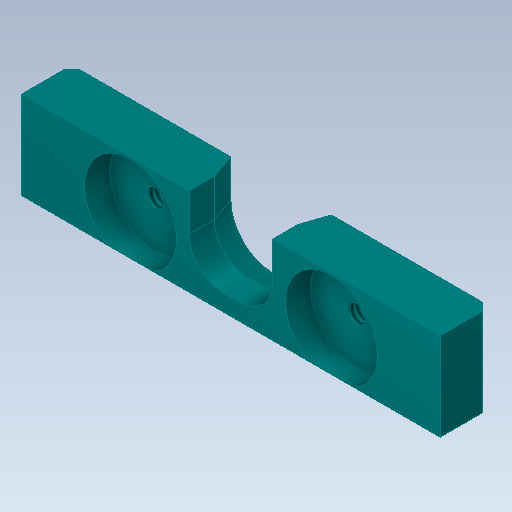
# Autodesk Inventor part: FAB-OX0021
Saved by Autodesk Inventor 2020 (Build 240168000, 168)
## iProperties
Created: 2017-02-10
Part Number: FAB-OX0021
Material: Aluminum 6061
Document SubType Name: Modeling
Designer: map
Density: 2.7 g/cm^3
Appearance: Anodized - Light Gray(1)
Description: Piezer pusher plate with cutout
Author: map
Revision Number: 01
Autodesk Inventor part; units mm, degrees
ref_plane "YZ Plane" through (0, 0, 0) normal (1, 0, 0) x (0, 1, 0)
ref_plane "XZ Plane" through (0, 0, 0) normal (0, 1, 0) x (-1, 0, 0)
ref_plane "XY Plane" through (0, 0, 0) normal (0, 0, 1) x (1, 0, 0)
derived "FAB-OX0020-PiezoPusher-Counter-Base.ipt"
sketch "Sketch1" plane through (0, 0, 0) normal (0, 1, 0) x (-1, 0, 0)
  line L0 (-25, -3) -> (25, -3)
  line L1 (25, -3) -> (25, 3)
  line L2 (25, 3) -> (-25, 3)
  line L3 (-25, 3) -> (-25, -3)
  line L4 (-25, -3) -> (25, 3) construction
  line L5 (25, -3) -> (-25, 3) construction
  point P0 (0, 0)
  dimension "d0" = 50
  dimension "d1" = 6
  constraints: 12 end point, 2 midpoint, 2 parallel, 1 horizontal, 1 perpendicular
  measures "d0" distance of L2.end L1.end
  measures "d1" distance of L1.end L0.end
extrude "Extrusion1" add sketch "Sketch1" against normal blind 11.5
sketch "Sketch2" plane through (-25, 0, 3) normal (0, 0, 1) x (1, 0, 0)
  line L0 (25, 0) -> (25, -11.5)
  line L1 (0, -11.5) -> (50, -11.5) projected
  line L2 (0, 0) -> (0, -11.5) projected
  line L3 (0, -5.75) -> (50, -5.75)
  line L4 (50, 0) -> (50, -11.5) projected
  point P0 (13, -5.75)
  point P1 (37, -5.75)
  dimension "d5" = 24
  constraints: 4 end point, 3 midpoint, 2 point on line, 1 symmetric about line
  measures "d5" distance of point (37, -5.75) point (13, -5.75)
hole "Hole1" at (-12, -5.75, 3) at (12, -5.75, 3) direction (0, 0, -1) diameter 2.156 depth 8.865 tip angle 118 counterbore diameter 11 counterbore depth 3 thread size "4-40 UNC" class "2B" standard "ANSI Unified Screw Threads"
sketch "Sketch5" plane through (-25, 0, 3) normal (0, 0, 1) x (1, 0, 0)
  line L0 (20, 0) -> (30, 0)
  line L1 (30, 0) -> (30, -8.5)
  line L2 (20, -8.5) -> (20, 0)
  line L3 (0, 0) -> (50, 0) projected
  line L4 (25, 0) -> (25, -3.5)
  line L5 (30, -8.5) -> (20, -8.5)
  dimension "d22" = 10
  dimension "d26" = 3.5
  dimension "d27" = 8.5
  constraints: 10 end point, 2 midpoint, 2 parallel, 1 horizontal, 1 perpendicular, 1 vertical
  measures "d22" distance of L0.start L0.end
  measures "d26" distance from line of L0 L4.end
  measures "d27" distance between parallel lines of L0 L5
extrude "Extrusion3" cut sketch "Sketch5" against normal through all
fillet "Fillet1" radius 4 2 edges at (-5, -8.5, 0) (5, -8.5, 0)
chamfer "Chamfer1" distance 1 angle 45 6 edges at (-25, -11.5, 0) (25, -11.5, 0) (0, -11.5, -3) (25, -5.75, -3) (-25, -5.75, -3) (0, -11.5, 3)
chamfer "Chamfer2" distance 1 distance2 3 5 edges at (0, -8.5, -3) (3.8284, -7.3284, -3) (5, -2.25, -3) (-3.8284, -7.3284, -3) (-5, -2.25, -3) measured on face at (4.182, -7.682, -3) measured on face at (-5.5, -2.25, -3) measured on face at (0, -9, -3) measured on face at (5.5, -2.25, -3) measured on face at (-4.182, -7.682, -3)
equation "\"d5\" = shaftSeparation"
equation "\"shaftSeparation\" = 24"
body "Solid1"
